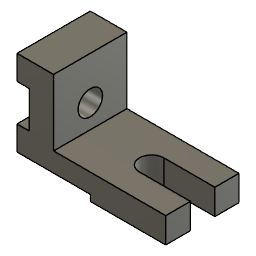
exv2_aug26 (Autodesk Fusion 360 design; units mm, degrees)
part number: 2026-08-27-22-24-47-787
Autodesk Fusion 360 part; units mm, degrees
sketch "Sketch2" plane through (0, 0, 0) normal (0, 1, 0) x (1, 0, 0)
  line L0 (730, 360) -> (-730, 360)
  line L1 (-730, 360) -> (-730, -360)
  line L2 (-730, -360) -> (730, -360)
  line L3 (730, -360) -> (730, 360)
  line L4 (730, 360) -> (-730, -360) construction
  line L5 (-730, 360) -> (730, -360) construction
  line L6 (-730, -360) -> (-10, -360)
  line L7 (-10, -360) -> (-10, 140)
  line L8 (-10, 140) -> (-730, 140)
  line L9 (-730, 140) -> (-730, -360)
  line L10 (230, 2.3053) -> (230, 122.3053)
  line L11 (230, 122.3053) -> (730, 122.3053)
  line L12 (230, -117.6947) -> (730, -117.6947)
  arc A0 (245.8705, 121.2512) -> (238.1032, -117.4208) centre (230, 2.3053) ccw
  dimension "d7" = 1460
  dimension "d8" = 720
  dimension "d9" = 720
  dimension "d10" = 500
  dimension "d11" = 240
  dimension "d12" = 500
  dimension "d13" = 90
  constraint horizontal L0
  constraint perpendicular L0 L1
  constraint parallel L0 L2
  constraint parallel L1 L3
  constraint coincident L4 origin
  constraint coincident L5 origin
  constraint horizontal L6
  constraint vertical L7
  constraint horizontal L8
  constraint vertical L9
  constraint coincident L10.start A0.centre
  constraint coincident L10.end A0
  constraint perpendicular L8 L10
  constraint coincident L12.start A0
  constraint tangent L12 A0
  constraint perpendicular L3 L12
  constraint coincident L3 L12.end
  constraint coincident L3 L11.end
  constraint coincident L5 A0.end
  constraint coincident L4 A0.start
  measures "d7" distance of L1.end L2.end
  measures "d8" distance of L0.end L1.end
  measures "d9" distance of L1.end L6.end
  measures "d10" distance of L1.end L8.end
  measures "d11" diameter of A0
  measures "d12" distance of L3 L10.start
  measures "d13" angle of L10 L11
extrude "Extrude1" add sketch "Sketch2" along normal blind 250 contours L0 L1 L2 L3 L7 L8 L11 L12 A0 | L1 L2 L6 L7 L8 L9
extrude "Extrude2" cut sketch "Sketch2" along normal blind 60 contours L1 L2 L6 L7 L8 L9
sketch "Sketch3" plane through (0, 250, 0) normal (0, 1, 0) x (-1, 0, 0)
  arc A0 (-230, -122.3053) -> (-230, 117.6947) centre (-230, -2.3053) ccw
  line L0 (-230, -122.3053) -> (-730, -122.3053)
  line L1 (-730, -122.3053) -> (-730, -360)
  line L2 (-730, -360) -> (730, -360)
  line L3 (730, -360) -> (730, 360)
  line L4 (730, 360) -> (-730, 360)
  line L5 (-730, 360) -> (-730, 117.6947)
  line L6 (-730, 117.6947) -> (-230, 117.6947)
  line L7 (730, 360) -> (370, 360)
  line L8 (370, 360) -> (370, -360)
  line L9 (370, -360) -> (730, -360)
  line L10 (730, -360) -> (730, 360)
  dimension "d18" = 360
  constraint horizontal L7
  constraint vertical L8
  constraint horizontal L9
  constraint vertical L10
  constraint coincident L2 L8.end
  constraint coincident L3.end L4.start
  measures "d18" distance of L3.end L7.end
extrude "Extrude3" add sketch "Sketch3" along normal blind 650 contours L2 L3 L4 L7 L8 L9 L10
sketch "Sketch4" plane through (-730, 0, 0) normal (-1, 0, 0) x (0, 0, 1)
  line L0 (-140, 0) -> (-140, 60)
  line L1 (-140, 60) -> (360, 60)
  line L2 (360, 60) -> (360, 900)
  line L3 (360, 900) -> (-360, 900)
  line L4 (-360, 900) -> (-360, 0)
  line L5 (-360, 0) -> (-140, 0)
  circle A0 centre (0, 480) radius 120
  circle A1 centre (0, 480) radius 300
  line L6 (-360, 900) -> (360, 900)
  line L7 (360, 900) -> (360, 660)
  line L8 (360, 660) -> (-360, 660)
  line L9 (-360, 660) -> (-360, 900)
  line L10 (360, 60) -> (-360, 60)
  line L11 (-360, 60) -> (-360, 300)
  line L12 (-360, 300) -> (360, 300)
  line L13 (360, 300) -> (360, 60)
  dimension "d21" = 240
  dimension "d22" = 600
  dimension "d23" = 480
  dimension "d24" = 240
  dimension "d25" = 240
  constraint concentric A0 A1
  constraint horizontal L6
  constraint vertical L7
  constraint horizontal L8
  constraint vertical L9
  constraint coincident L2 L7.end
  constraint coincident L3.end L4.start
  constraint horizontal L10
  constraint vertical L11
  constraint horizontal L12
  constraint vertical L13
  constraint coincident L4 L11.end
  constraint coincident L1.end L2.start
  measures "d21" diameter of A0
  measures "d22" diameter of A1
  measures "d23" distance of L5 A0.centre
  measures "d24" distance of L2.end L7.end
  measures "d25" distance of L1.end L12.end
extrude "Extrude4" cut sketch "Sketch4" against normal through all contours A0
extrude "Extrude5" cut sketch "Sketch4" against normal blind 120 contours L2 A1 L8 L12 | L4 A1 L8 L12 | A1 L8 L12 | A1 L12 | A1 L8
